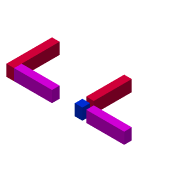
# Autodesk Inventor part: CellDecompExample
Saved by Autodesk Inventor 2014 (Build 180170000, 170)
## iProperties
Created: 2015-07-28
Part Number: CellDecompExample
Material: Generic
Document SubType Name: Modeling
Designer: kulkarni
Density: 1 g/cm^3
Appearance: Default
Author: kulkarni
Autodesk Inventor part; units mm, degrees
ref_plane "YZ Plane" through (0, 0, 0) normal (1, 0, 0) x (0, 1, 0)
ref_plane "XZ Plane" through (0, 0, 0) normal (0, 1, 0) x (-1, 0, 0)
ref_plane "XY Plane" through (0, 0, 0) normal (0, 0, 1) x (1, 0, 0)
sketch "Sketch1" plane through (0, 0, 0) normal (0, 0, 1) x (1, 0, 0)
  line L0 (0, 120) -> (20, 120)
  line L1 (20, 120) -> (20, 0)
  line L2 (20, 0) -> (0, 0)
  line L3 (0, 0) -> (0, 120)
  line L4 (120, 0) -> (20, 0)
  line L5 (20, 0) -> (20, 20)
  line L6 (20, 20) -> (120, 20)
  line L7 (120, 20) -> (120, 0)
  line L8 (180, 120) -> (200, 120)
  line L9 (200, 120) -> (200, 20)
  line L10 (200, 20) -> (180, 20)
  line L11 (180, 20) -> (180, 120)
  line L12 (180, 20) -> (200, 20)
  line L13 (200, 20) -> (200, 0)
  line L14 (200, 0) -> (180, 0)
  line L15 (180, 0) -> (180, 20)
  line L16 (200, 20) -> (300, 20)
  line L17 (300, 20) -> (300, 0)
  line L18 (300, 0) -> (200, 0)
  line L19 (200, 0) -> (200, 20)
  constraints: 40 end point, 10 parallel, 5 horizontal, 5 perpendicular, 1 point on line
extrude "Extrusion1" add sketch "Sketch1" along normal blind 30 contours L0 L1 L2 L3
extrude "Extrusion2" add sketch "Sketch1" along normal blind 30 separate body contours L6 L7 L4 L1
extrude "Extrusion3" add sketch "Sketch1" along normal blind 30 separate body contours L8 L9 L10 L11
extrude "Extrusion4" add sketch "Sketch1" along normal blind 30 separate body contours L10 L13 L14 L15
extrude "Extrusion5" add sketch "Sketch1" along normal blind 30 separate body contours L16 L17 L18 L13
move or copy body "Move Body1" bodies to move or copy 3 copy no translate (0, 10, 0)
move or copy body "Move Body2" bodies to move or copy 5 copy no translate (10, 0, 0)
body "Solid1"
body "Solid2"
body "Solid3"
body "Solid4"
body "Solid5"
